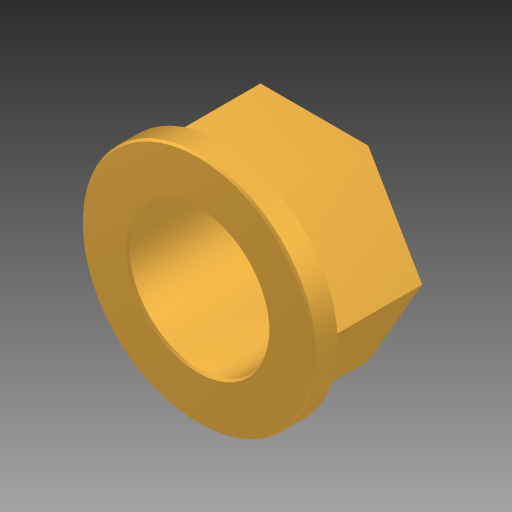
# Autodesk Inventor part: WCP 500 Hex Bushing
Saved by Autodesk Inventor 2023 (Build 270158000, 158)
## iProperties
Created: 2022-12-17
Part Number: WCP 500 Hex Bushing
Material: Brass, Soft Yellow
Document SubType Name: Modeling
Designer: Max Boord
Mass: 5.37809 g
Surface Area: 8.43472 cm^2
Volume: 0.634958 cm^3
Density: 8.47 g/cm^3
Appearance: Brass - Satin
Author: Max Boord
Autodesk Inventor part; units mm, degrees
ref_plane "YZ Plane" through (0, 0, 0) normal (1, 0, 0) x (0, 1, 0)
ref_plane "XZ Plane" through (0, 0, 0) normal (0, 1, 0) x (-1, 0, 0)
ref_plane "XY Plane" through (0, 0, 0) normal (0, 0, 1) x (1, 0, 0)
sketch "Sketch1" plane through (0, 0, 0) normal (1, 0, 0) x (0, 1, 0)
  line L0 (0, 0) -> (4.7625, 0)
  line L1 (4.7625, 0) -> (4.7625, 1.5875)
  line L2 (4.7625, 1.5875) -> (7.9375, 1.5875)
  line L3 (7.9375, 1.5875) -> (7.9375, 0)
  line L4 (7.9375, 0) -> (6.35, 0)
  line L5 (6.35, 0) -> (6.35, -6.35)
  line L6 (6.35, -6.35) -> (4.7625, -6.35)
  line L7 (4.7625, -6.35) -> (4.7625, 0)
  line L8 (0, 0) -> (0, -7.0209)
  dimension "d0" = 9.525
  dimension "d1" = 12.7
  dimension "d2" = 15.875
  dimension "d3" = 1.5875
  dimension "d4" = 6.35
  constraints: 18 end point, 6 perpendicular, 3 point on line, 1 horizontal, 1 vertical
  measures "d0" diameter of L7 L8
  measures "d1" diameter of L5 L8
  measures "d2" diameter of L3 L8
  measures "d3" distance between parallel lines of L4 L2
  measures "d4" distance of L4.end L5.end
revolve "Revolution1" add sketch "Sketch1" angle 360 about axis through (0, 0, 0) along (0, 0, -1)
sketch "Sketch2" plane through (0, 0, -6.35) normal (0, 0, -1) x (-1, 0, 0)
  circle A0 centre (0, 0) radius 6.35 projected
  line L0 (-7.3323, 0) -> (-3.6662, 6.35)
  line L1 (-3.6662, 6.35) -> (3.6662, 6.35)
  line L2 (3.6662, 6.35) -> (7.3323, 0)
  line L3 (7.3323, 0) -> (3.6662, -6.35)
  line L4 (3.6662, -6.35) -> (-3.6662, -6.35)
  line L5 (-3.6662, -6.35) -> (-7.3323, 0)
  point P0 (-5.4993, -3.175)
  point P1 (0, -6.35)
  point P2 (-5.4993, 3.175)
  point P3 (5.4993, -3.175)
  point P4 (5.4993, 3.175)
  point P5 (0, 6.35)
  constraints: 12 end point, 1 coincident, 1 horizontal, 1 tangent, 13 other
extrude "Extrusion1" add sketch "Sketch2" against normal up to surface (6.35 mm away) contours A0 L2 L3 | A0 L1 L2 | L3 L4 A0 | A0 L0 L1 | L4 L5 A0 | A0 L5 L0
chamfer "Chamfer1" distance 0.127 angle 45 2 edges at (0, -7.9375, 1.5875) (0, -4.7625, 1.5875)
body "Solid1"
